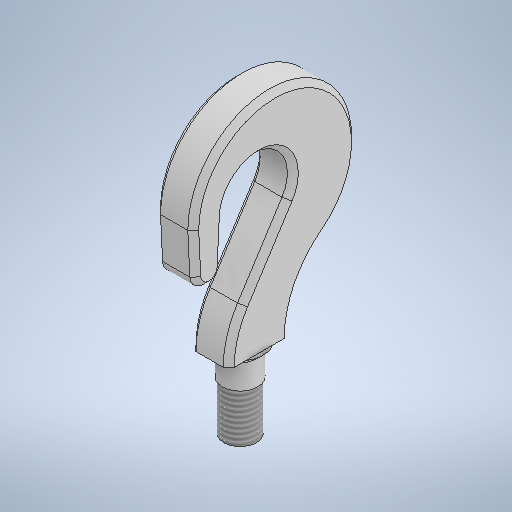
# Autodesk Inventor part: Gancho
Saved by Autodesk Inventor 2025.3 (Build 293356030, 356C)
## iProperties
Created: 2025-08-24
Part Number: Gancho
Material: Generic
Document SubType Name: Modeling
Designer: PC
Density: 1 g/cm^3
Appearance: Default
Author: PC
Autodesk Inventor part; units mm, degrees
ref_plane "YZ Plane" through (0, 0, 0) normal (1, 0, 0) x (0, 1, 0)
ref_plane "XZ Plane" through (0, 0, 0) normal (0, 1, 0) x (-1, 0, 0)
sketch "Sketch1" plane through (0, 0, 0) normal (1, 0, 0) x (0, 1, 0)
  arc A0 (26.1895, -3.5687) -> (0, 9.3537) centre (0, -23.6463) ccw
  arc A1 (17.8047, 26.4685) -> (0, 31.6837) centre (0, -1.3163) ccw
  line L0 (91.8773, 20.6837) -> (-78.3169, 20.6837)
  arc A2 (43.2558, 10.1592) -> (50, 33.1837) centre (50, 20.6837) ccw
  arc A3 (26.1895, -3.5687) -> (50, 44.6837) centre (49.9981, 14.6837) ccw
  line L1 (43.2558, 10.1592) -> (17.8047, 26.4685)
  line L2 (0, 54.8963) -> (0, -73.9166)
  line L3 (50, 20.6837) -> (50, 74.3533) construction
  line L4 (50, 44.6837) -> (50, 33.1837)
  arc A4 (34.7544, 43.9339) -> (34.7503, 33.9462) centre (35, 38.94) ccw
  line L5 (50, 44.6837) -> (34.7544, 43.9339)
  line L6 (50, 33.1837) -> (34.7503, 33.9462)
  point P0 (0, 0)
  point P1 (0, 20.6837)
  dimension "d0" = 66
  dimension "d1" = 66
  dimension "d2" = 22.33
  dimension "d3" = 22
  dimension "d4" = 25
  dimension "d5" = 50
  dimension "d6" = 60
  dimension "d7" = 6
  dimension "d8" = 10
  dimension "d9" = 15
  constraints: 14 end point, 10 point on circle, 6 point on line, 5 centre point, 5 tangent, 2 vertical, 1 collinear, 1 horizontal
  measures "d0" diameter of A0
  measures "d1" diameter of A1
  measures "d2" distance of A0.centre A1.centre
  measures "d3" distance of A1.centre point (0, 20.684)
  measures "d4" diameter of A2
  measures "d5" horizontal distance of A1.centre L3.start
  measures "d6" diameter of A3
  measures "d7" distance of A3.centre L3.start
  measures "d8" diameter of A4
  measures "d9" distance from line of A4.centre L4
extrude "Extrusion1" add sketch "Sketch1" along normal blind 14 contours A0 L2 L0 L1 A2 A3 | L0 A2 L4 A3 | L2 A1 L1 L0 | L4 L6 A4 L5
chamfer "Chamfer1" distance 2 angle 45 16 edges at (14, 76.901, 1.4083) (14, 14.602, 5.9473) (0, 76.901, 1.4083) (0, 14.602, 5.9473) (14, 42.3752, 33.565) (14, 30, 38.942) (14, 42.3772, 44.3088) (14, 61.996, 17.1699) (14, 30.5303, 18.3138) (14, 9.2764, 30.3531) (0, 42.3772, 44.3088) (0, 30, 38.942) (0, 42.3752, 33.565) (0, 30.5303, 18.3138) (0, 9.2764, 30.3531) (0, 61.996, 17.1699)
ref_plane "Work Plane1" through (7, 0, 0) normal (-1, 0, 0) x (0, 0, 1)
sketch "Sketch2" plane through (7, 0, 0) normal (-1, 0, 0) x (0, 0, 1)
  line L0 (29.6837, 0) -> (11.3537, 0) projected
  line L1 (26.5187, 0) -> (14.5187, 0)
  line L2 (26.5187, -29) -> (26.5187, -11.0524)
  line L3 (27.0187, -11.0524) -> (27.0187, -2)
  line L4 (29.0187, 0) -> (30.2528, 0)
  line L5 (12.0186, 0) -> (11.3537, 0)
  arc A0 (29.0187, 0) -> (27.0187, -2) centre (29.0187, -2) ccw
  line L6 (20.5187, -31.2918) -> (20.5187, 0)
  line L7 (29.0187, 0) -> (12.0186, 0)
  line L8 (27.0187, -11.0524) -> (26.5187, -11.0524)
  arc A1 (20.5187, -31.2918) -> (26.5187, -29) centre (20.7329, -22.8528) ccw
  line L9 (29.0187, 0) -> (20.5187, 0)
  point P0 (0, 0)
  point P1 (27.0187, 0)
  dimension "d19" = 0.5
  dimension "d20" = 2
  dimension "d21" = 6
  dimension "d22" = 31.2918
  constraints: 18 end point, 4 point on circle, 4 point on line, 4 tangent, 3 coincident, 3 collinear, 3 midpoint, 2 centre point, 2 perpendicular, 1 horizontal, 1 vertical
  measures "d19" distance from line of L2 L3.start
  measures "d20" radius of A0
  measures "d21" horizontal distance of L2.start A1.start
  measures "d22" distance of L9.end A1.start
revolve "Revolution1" add sketch "Sketch2" angle 360 about axis through (7, -31.2918, 20.5187) along (0, 1, 0)
thread "Thread1" size "M12x1.75" class "6g" standard "ISO Metric profile" length 13
thread "Thread2" size "M12x1.75" class "6g" standard "ANSI Metric M Profile" length 13
body "Solid1"
